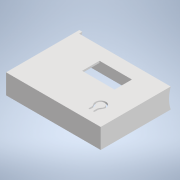
# Autodesk Inventor part: tacho_base
Saved by Autodesk Inventor 2022 (Build 260153000, 153)
## iProperties
Created: 2024-07-12
Part Number: tacho_base
Material: Типовые
Document SubType Name: Modeling
Designer: Капустяник Андрей
Density: 1 g/cm^3
Appearance: По умолчанию
Author: Капустяник Андрей
Autodesk Inventor part; units mm, degrees
ref_plane "YZ Plane" through (0, 0, 0) normal (1, 0, 0) x (0, 1, 0)
ref_plane "XZ Plane" through (0, 0, 0) normal (0, 1, 0) x (-1, 0, 0)
ref_plane "XY Plane" through (0, 0, 0) normal (0, 0, 1) x (1, 0, 0)
sketch "Эскиз1" plane through (0, 0, 0) normal (0, 1, 0) x (-1, 0, 0)
  line L0 (50, -40) -> (-50, -40)
  line L1 (-50, -40) -> (-50, 40)
  line L2 (-50, 40) -> (50, 40)
  line L3 (50, 40) -> (50, -40)
  line L4 (50, -40) -> (-50, 40) construction
  line L5 (-50, -40) -> (50, 40) construction
  line L6 (21.6, -30) -> (-21.6, -30)
  line L7 (-21.6, -30) -> (-21.6, -6.9)
  line L8 (-21.6, -6.9) -> (21.6, -6.9)
  line L9 (21.6, -6.9) -> (21.6, -30)
  line L10 (-53, -43) -> (53, -43)
  line L11 (53, -43) -> (53, 43)
  line L12 (53, 43) -> (-53, 43)
  line L13 (-53, 43) -> (-53, -43)
  line L14 (53, 43) -> (68, 43)
  line L15 (68, 43) -> (68, -43)
  line L16 (68, -43) -> (53, -43)
  line L17 (53, -43) -> (53, 43)
  line L18 (-53, -43) -> (68, -43)
  line L19 (68, -43) -> (68, 43)
  line L20 (68, 43) -> (-53, 43)
  line L21 (-53, 43) -> (-53, -43)
  line L22 (0, -40) -> (0, 40)
  circle A0 centre (-30, 20) radius 5
  circle A1 centre (-30, 20) radius 7
  line L23 (-30, 20) -> (-30, 40)
  line L24 (-28, 30.5826) -> (-32, 30.5826)
  line L25 (-32, 30.5826) -> (-32, 24.5826)
  line L26 (-32, 24.5826) -> (-28, 24.5826)
  line L27 (-28, 24.5826) -> (-28, 30.5826)
  line L28 (-28, 30.5826) -> (-32, 24.5826) construction
  line L29 (-32, 30.5826) -> (-28, 24.5826) construction
  line L30 (-34, 22.5826) -> (-34, 32.5826)
  line L31 (-34, 32.5826) -> (-26, 32.5826)
  line L32 (-26, 32.5826) -> (-26, 22.5826)
  line L33 (-26, 22.5826) -> (-34, 22.5826)
  line L34 (-28, 30.5826) -> (-32, 30.5826)
  line L35 (-32, 30.5826) -> (-32, 32.5826)
  line L36 (-32, 32.5826) -> (-28, 32.5826)
  line L37 (-28, 32.5826) -> (-28, 30.5826)
  line L38 (-55.5, -45.5) -> (70.5, -45.5)
  line L39 (70.5, -45.5) -> (70.5, 45.5)
  line L40 (-55.5, -45.5) -> (-55.5, 45.5)
  line L41 (-55.5, 45.5) -> (70.5, 45.5)
  point P0 (0, 0)
  point P1 (0, -30)
  point P2 (-30, 27.5826)
  point P3 (53, -43)
  point P4 (-26, 25.7446)
  point P5 (-34, 25.7446)
  point P6 (53, -43)
  dimension "d7" = 10
  dimension "d0" = 100
  dimension "d1" = 80
  dimension "d2" = 43.2
  dimension "d3" = 23.1
  dimension "d4" = 3
  dimension "d5" = 15
  dimension "d6" = 10
  dimension "d8" = 2
  dimension "d9" = 20
  dimension "d10" = 20
  dimension "d11" = 4
  dimension "d12" = 6
  dimension "d13" = 2
  dimension "d22" = 2.5
  dimension "d23" = 2.5
  constraints: 84 end point, 16 parallel, 10 perpendicular, 7 midpoint, 6 horizontal, 4 point on line, 2 collinear, 1 centre point, 11 other
  measures "d0" distance of L1.end L2.end
  measures "d1" distance of L0.end L1.end
  measures "d2" distance of L7.end L8.end
  measures "d3" distance of L6.end L7.end
  measures "d4" distance between parallel lines of L0 L10
  measures "d5" distance of L15.end L16.end
  measures "d6" distance between parallel lines of L0 L6
  measures "d9" distance from line of L2 L23.start
  measures "d10" distance from line of L1 L23.start
  measures "d11" distance of L26.end L25.end
  measures "d12" distance of L24.end L25.end
  measures "d13" distance between parallel lines of L25 L30
  measures "d22" distance between parallel lines of L18 L38
  measures "d23" distance between parallel lines of L21 L40
extrude "Выдавливание1" add sketch "Эскиз1" along normal blind 2.5 contours L0 L22 L6 L9 L8 L2 L3 | L0 L1 L2 L22 L8 L7 L6 | L13 L12 L11 L10 | L11 L14 L15 L16 | A0 L30 L33 L32 | L32 L33 L23 L26 A0 | A0 L26 L23 L33 L30 | L26 L23 A0 | A0 L23 A1 L27 | L25 A1 L23 A0 | A0 L23 L26 | A1 L23 L24 L27 | L25 L24 L23 A1 | L24 L23 L31 L37 | L35 L31 L23 L24 | L40 L41 L39 L38
fillet "Сопряжение1" radius 5 4 edges at (26, 1.25, 25.7446) (28, 1.25, 24.5826) (32, 1.25, 24.5826) (34, 1.25, 25.7446)
fillet "Сопряжение2" radius 1 4 edges at (26, 1.25, 32.5826) (28, 1.25, 32.5826) (32, 1.25, 32.5826) (34, 1.25, 32.5826)
sketch "Эскиз2" plane through (0, 0, 0) normal (0, -1, 0) x (1, 0, 0)
  line L0 (-21.6, -30) -> (21.6, -30) projected
  line L1 (-21.6, -6.9) -> (-21.6, -30) projected
  line L2 (21.6, -6.9) -> (-21.6, -6.9) projected
  line L3 (21.6, -30) -> (21.6, -6.9) projected
  arc A0 (34, 27.9373) -> (35.25, 24.6301) centre (39, 27.9373) ccw projected
  arc A1 (24.75, 24.6301) -> (35.25, 24.6301) centre (30, 20) ccw projected
  arc A2 (24.75, 24.6301) -> (26, 27.9373) centre (21, 27.9373) ccw projected
  line L4 (26, 31.5826) -> (26, 27.9373) projected
  arc A3 (28, 31.5826) -> (26, 31.5826) centre (27, 31.5826) ccw projected
  line L5 (28, 27.1414) -> (28, 31.5826) projected
  arc A4 (26.5, 23.5707) -> (28, 27.1414) centre (23, 27.1414) ccw projected
  arc A5 (26.5, 23.5707) -> (33.5, 23.5707) centre (30, 20) ccw projected
  arc A6 (32, 27.1414) -> (33.5, 23.5707) centre (37, 27.1414) ccw projected
  line L6 (32, 31.5826) -> (32, 27.1414) projected
  arc A7 (34, 31.5826) -> (32, 31.5826) centre (33, 31.5826) ccw projected
  line L7 (34, 27.9373) -> (34, 31.5826) projected
  circle A8 centre (30, 20) radius 2.5
  point P0 (0, 0)
  dimension "d18" = 5
  constraints: 1 centre point, 1 coincident
  measures "d18" diameter of A8
extrude "Выдавливание2" add sketch "Эскиз2" along normal blind 2.5 contours A8
fillet "Сопряжение3" radius 2 1 edges at (27.5, 0, 20)
sketch "Эскиз3" plane through (0, 0, 0) normal (0, -1, 0) x (1, 0, 0)
  arc A0 (34, 27.9373) -> (35.25, 24.6301) centre (39, 27.9373) ccw projected
  arc A1 (24.75, 24.6301) -> (35.25, 24.6301) centre (30, 20) ccw projected
  arc A2 (24.75, 24.6301) -> (26, 27.9373) centre (21, 27.9373) ccw projected
  line L0 (26, 31.5826) -> (26, 27.9373) projected
  arc A3 (28, 31.5826) -> (26, 31.5826) centre (27, 31.5826) ccw projected
  line L1 (28, 27.1414) -> (28, 31.5826) projected
  arc A4 (26.5, 23.5707) -> (28, 27.1414) centre (23, 27.1414) ccw projected
  arc A5 (26.5, 23.5707) -> (33.5, 23.5707) centre (30, 20) ccw projected
  arc A6 (32, 27.1414) -> (33.5, 23.5707) centre (37, 27.1414) ccw projected
  line L2 (32, 31.5826) -> (32, 27.1414) projected
  arc A7 (34, 31.5826) -> (32, 31.5826) centre (33, 31.5826) ccw projected
  line L3 (34, 27.9373) -> (34, 31.5826) projected
  line L4 (-21.6, -30) -> (21.6, -30) projected
  line L5 (-21.6, -6.9) -> (-21.6, -30) projected
  line L6 (21.6, -6.9) -> (-21.6, -6.9) projected
  line L7 (21.6, -30) -> (21.6, -6.9) projected
  circle A8 centre (30, 20) radius 4.5 projected
  line L8 (55.5, -45.5) -> (-70.5, -45.5) projected
  line L9 (55.5, 45.5) -> (55.5, -45.5) projected
  line L10 (-70.5, 45.5) -> (55.5, 45.5) projected
  line L11 (-70.5, -45.5) -> (-70.5, 45.5) projected
  arc A9 (34, 27.9373) -> (35.25, 24.6301) centre (39, 27.9373) ccw projected
  arc A10 (24.75, 24.6301) -> (35.25, 24.6301) centre (30, 20) ccw projected
  arc A11 (24.75, 24.6301) -> (26, 27.9373) centre (21, 27.9373) ccw projected
  line L12 (26, 31.5826) -> (26, 27.9373) projected
  arc A12 (28, 31.5826) -> (26, 31.5826) centre (27, 31.5826) ccw projected
  line L13 (28, 27.1414) -> (28, 31.5826) projected
  arc A13 (26.5, 23.5707) -> (28, 27.1414) centre (23, 27.1414) ccw projected
  arc A14 (26.5, 23.5707) -> (33.5, 23.5707) centre (30, 20) ccw projected
  arc A15 (32, 27.1414) -> (33.5, 23.5707) centre (37, 27.1414) ccw projected
  line L14 (32, 31.5826) -> (32, 27.1414) projected
  arc A16 (34, 31.5826) -> (32, 31.5826) centre (33, 31.5826) ccw projected
  line L15 (34, 27.9373) -> (34, 31.5826) projected
  line L16 (-21.6, -30) -> (21.6, -30) projected
  line L17 (-21.6, -6.9) -> (-21.6, -30) projected
  line L18 (21.6, -6.9) -> (-21.6, -6.9) projected
  line L19 (21.6, -30) -> (21.6, -6.9) projected
  circle A17 centre (30, 20) radius 4.5 projected
  line L20 (53, 43) -> (53, -43)
  line L21 (53, -43) -> (-68, -43)
  line L22 (-68, -43) -> (-68, 43)
  line L23 (-68, 43) -> (53, 43)
  dimension "d28" = 2.5
  constraints: 8 end point, 3 other
  measures "d28" distance between parallel lines of L10 L23
extrude "Выдавливание3" add sketch "Эскиз3" along normal blind 24.04 contours L8 L11 L10 L9
sketch "Эскиз4" plane through (-70.5, 2.5, -45.5) normal (-1, 0, 0) x (0, 0, 1)
  line L0 (91, -26.54) -> (91, 0) projected
  line L1 (0, 0) -> (91, 0) projected
  line L2 (0, -26.54) -> (0, 0) projected
  line L3 (91, -26.54) -> (0, -26.54) projected
  line L4 (0, 0) -> (0, -26.54) projected
  line L5 (0, -13.27) -> (-40, -13.27)
  circle A0 centre (-40, -13.27) radius 40
  line L6 (0, -26.54) -> (0, 0) projected
  line L7 (0, -26.54) -> (-2.2653, -26.54)
  line L8 (-2.2653, -26.54) -> (-2.2653, 0)
  line L9 (-2.2653, 0) -> (0, 0)
  line L10 (0, 0) -> (0, -26.54)
  line L11 (0, 0) -> (91, 0) projected
  point P0 (45.5, -2.5)
  point P1 (-2.2653, -26.54)
  dimension "d29" = 80
  constraints: 10 end point, 2 horizontal, 2 parallel, 1 coincident, 1 collinear, 1 midpoint, 1 perpendicular, 1 vertical, 3 other
extrude "Выдавливание4" add sketch "Эскиз4" against normal up to surface (126 mm away) contours L7 A0 L2 | L2 A0 L9
sketch "Эскиз5" plane through (-70.5, -24.04, 45.5) normal (-1, 0, 0) x (0, 0, 1)
  line L0 (0, 0) -> (0, 26.54) projected
  line L1 (0, 26.54) -> (-93.2653, 26.54) projected
  arc A0 (-93.2653, 0) -> (-93.2653, 26.54) centre (-131, 13.27) ccw projected
  line L2 (0, 0) -> (-93.2653, 0) projected
  circle A1 centre (-131, 13.27) radius 40
  circle A2 centre (-131, 13.27) radius 36
  line L3 (-93.2653, 0) -> (-97.535, 0)
  arc A3 (-93.2653, 0) -> (-93.2653, 26.54) centre (-131, 13.27) ccw projected
  line L4 (-93.2653, 26.54) -> (-97.535, 26.54)
  point P0 (-45.5, 24.04)
  dimension "d32" = 4
  constraints: 4 end point, 2 centre point, 2 point on circle, 1 coincident, 1 concentric, 1 horizontal, 1 parallel
  measures "d32" radial gap between concentric circles of A1 A2
extrude "Выдавливание5" add sketch "Эскиз5" against normal blind 4 contours L3 A2 L4 A0
